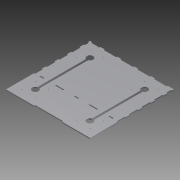
# Autodesk Inventor part: base top2
Saved by Autodesk Inventor 2011 (Build 150239000, 239)
## iProperties
Created: 2011-07-30
Part Number: base top2
Document SubType Name: Modeling
Designer: adowning
Density: 1 g/cm^3
Author: adowning
Autodesk Inventor part; units mm, degrees
(part 1 of 2)
ref_plane "YZ Plane" through (0, 0, 0) normal (1, 0, 0) x (0, 1, 0)
ref_plane "XZ Plane" through (0, 0, 0) normal (0, 1, 0) x (-1, 0, 0)
ref_plane "XY Plane" through (0, 0, 0) normal (0, 0, 1) x (1, 0, 0)
sketch "Sketch1" plane through (0, 0, 0) normal (0, 0, 1) x (1, 0, 0)
  point P0 (0, 0)
sketch "Sketch2" plane through (0, 0, 0) normal (0, 1, 0) x (-1, 0, 0)
  line L0 (74.6367, 49.7732) -> (-433.3633, 49.7732)
  line L1 (-433.3633, 49.7732) -> (-433.3633, -458.2268)
  line L2 (-433.3633, -458.2268) -> (74.6367, -458.2268)
  line L3 (74.6367, -458.2268) -> (74.6367, 49.7732)
  line L4 (74.6367, -458.2268) -> (-14.2633, -458.2268)
  line L5 (-14.2633, -382.0268) -> (-14.2633, -369.3268)
  line L6 (-14.2633, -369.3268) -> (-1.5633, -369.3268)
  line L7 (74.6367, -369.3268) -> (74.6367, -458.2268)
  line L8 (-433.3633, -458.2268) -> (-344.4633, -458.2268)
  line L9 (-344.4633, -382.0268) -> (-344.4633, -369.3268)
  line L10 (-344.4633, -369.3268) -> (-357.1633, -369.3268)
  line L11 (-433.3633, -369.3268) -> (-433.3633, -458.2268)
  line L12 (-433.3633, 49.7732) -> (-344.4633, 49.7732)
  line L13 (-344.4633, -26.4268) -> (-344.4633, -39.1268)
  line L14 (-344.4633, -39.1268) -> (-357.1633, -39.1268)
  line L15 (-433.3633, -39.1268) -> (-433.3633, 49.7732)
  line L16 (74.6367, 49.7732) -> (-14.2633, 49.7732)
  line L17 (-14.2633, -26.4268) -> (-14.2633, -39.1268)
  line L18 (-14.2633, -39.1268) -> (-1.5633, -39.1268)
  line L19 (74.6367, -39.1268) -> (74.6367, 49.7732)
  line L20 (74.6367, -458.2268) -> (26.0973, -458.2268)
  line L21 (26.0973, -411.6686) -> (26.0973, -409.6874)
  line L22 (26.0973, -409.6874) -> (28.0785, -409.6874)
  line L23 (74.6367, -409.6874) -> (74.6367, -458.2268)
  line L24 (-433.3633, 49.7732) -> (-384.8239, 49.7732)
  line L25 (-384.8239, 49.7732) -> (-384.8239, 5.3232)
  line L26 (-384.8239, 5.3232) -> (-433.3633, 5.3232)
  line L27 (-433.3633, 5.3232) -> (-433.3633, 49.7732)
  line L28 (74.6367, -458.2268) -> (-54.6239, -458.2268)
  line L29 (74.6367, -328.9662) -> (74.6367, -458.2268)
  line L30 (-433.3633, 49.7732) -> (-304.1027, 49.7732)
  line L31 (-433.3633, -79.4874) -> (-433.3633, 49.7732)
  line L32 (-433.3633, 49.7732) -> (-384.8239, 49.7732)
  line L33 (-384.8239, 1.2338) -> (-386.8051, 1.2338)
  line L34 (-433.3633, 1.2338) -> (-433.3633, 49.7732)
  circle A0 centre (26.0973, -409.6874) radius 1.9812
  circle A1 centre (-54.6239, -409.6874) radius 1.9812
  circle A2 centre (-54.6239, -328.9662) radius 1.9812
  circle A3 centre (26.0973, -328.9662) radius 1.9812
  circle A4 centre (-304.1027, -409.6874) radius 1.9812
  arc A5 (-386.8051, -409.6874) -> (-384.8239, -407.7062) centre (-384.8239, -409.6874) ccw
  circle A6 centre (-384.8239, -328.9662) radius 1.9812
  circle A7 centre (-304.1027, -328.9662) radius 1.9812
  circle A8 centre (-304.1027, -79.4874) radius 1.9812
  circle A9 centre (-384.8239, -79.4874) radius 1.9812
  circle A10 centre (-384.8239, 1.2338) radius 1.9812
  circle A11 centre (-304.1027, 1.2338) radius 1.9812
  circle A12 centre (26.0973, 1.2338) radius 1.9812
  circle A13 centre (26.0973, -79.4874) radius 1.9812
  circle A14 centre (-54.6239, -79.4874) radius 1.9812
  circle A15 centre (-54.6239, 1.2338) radius 1.9812
  circle A16 centre (-14.2633, -369.3268) radius 12.7
  circle A17 centre (-344.4633, -369.3268) radius 12.7
  circle A18 centre (-344.4633, -39.1268) radius 12.7
  circle A19 centre (-14.2633, -39.1268) radius 12.7
  line L35 (26.0973, -409.6874) -> (26.0973, -407.7062)
  line L36 (26.0973, -409.6874) -> (24.1161, -409.6874)
  line L37 (-54.6239, -328.9662) -> (-52.6427, -328.9662)
  line L38 (24.1161, -328.9662) -> (28.0785, -328.9662)
  line L39 (26.0973, -330.9474) -> (26.0973, -326.985)
  line L40 (-54.6239, -328.9662) -> (-54.6239, -326.985)
  line L41 (-54.6239, -411.6686) -> (-54.6239, -407.7062)
  line L42 (-54.6239, -330.9474) -> (-54.6239, -328.9662)
  line L43 (-54.6239, -328.9662) -> (-56.6051, -328.9662)
  line L44 (-52.6427, -409.6874) -> (-56.6051, -409.6874)
  line L45 (-302.1215, -409.6874) -> (-306.0839, -409.6874)
  line L46 (-382.8427, -409.6874) -> (-386.8051, -409.6874)
  line L47 (-384.8239, -407.7062) -> (-384.8239, -411.6686)
  line L48 (-302.1215, -328.9662) -> (-306.0839, -328.9662)
  line L49 (-382.8427, -328.9662) -> (-386.8051, -328.9662)
  line L50 (-384.8239, -326.985) -> (-384.8239, -330.9474)
  line L51 (-304.1027, -407.7062) -> (-304.1027, -411.6686)
  line L52 (-304.1027, -79.4874) -> (-304.1027, -81.4686)
  line L53 (-304.1027, -326.985) -> (-304.1027, -330.9474)
  line L54 (-384.8239, 1.2338) -> (-382.8427, 1.2338)
  line L55 (-384.8239, 1.2338) -> (-384.8239, -0.7474)
  line L56 (-384.8239, -77.5062) -> (-384.8239, -81.4686)
  line L57 (-304.1027, -79.4874) -> (-306.0839, -79.4874)
  line L58 (-382.8427, -79.4874) -> (-386.8051, -79.4874)
  line L59 (-384.8239, 49.7732) -> (-384.8239, 5.3232)
  line L60 (-384.8239, 3.215) -> (-384.8239, 1.2338)
  line L61 (-304.1027, 3.215) -> (-304.1027, -0.7474)
  line L62 (-304.1027, -77.5062) -> (-304.1027, -79.4874)
  line L63 (-306.0839, 1.2338) -> (-302.1215, 1.2338)
  line L64 (-304.1027, -79.4874) -> (-302.1215, -79.4874)
  line L65 (-56.6051, -79.4874) -> (-52.6427, -79.4874)
  line L66 (24.1161, -79.4874) -> (28.0785, -79.4874)
  line L67 (-54.6239, -81.4686) -> (-54.6239, -77.5062)
  line L68 (-54.6239, -0.7474) -> (-54.6239, 3.215)
  line L69 (-56.6051, 1.2338) -> (-52.6427, 1.2338)
  line L70 (24.1161, 1.2338) -> (28.0785, 1.2338)
  line L71 (26.0973, -81.4686) -> (26.0973, -77.5062)
  line L72 (26.0973, -0.7474) -> (26.0973, 3.215)
  point P0 (0, 0)
  dimension "d0" = 508
  dimension "d1" = 508
  dimension "d2" = 88.9
  dimension "d3" = 88.9
  dimension "d4" = 88.9
  dimension "d5" = 88.9
  dimension "d6" = 88.9
  dimension "d7" = 88.9
  dimension "d8" = 88.9
  dimension "d9" = 88.9
  dimension "d10" = 48.5394
  dimension "d11" = 48.5394
  dimension "d12" = 48.5394
  dimension "d13" = 129.2606
  dimension "d14" = 129.2606
  dimension "d15" = 129.2606
  dimension "d16" = 129.2606
  dimension "d17" = 48.5394
  dimension "d18" = 48.5394
  dimension "d19" = 3.9624
  dimension "d20" = 3.9624
  dimension "d21" = 3.9624
  dimension "d22" = 3.9624
  dimension "d23" = 3.9624
  dimension "d24" = 3.9624
  dimension "d25" = 3.9624
  dimension "d26" = 3.9624
  dimension "d27" = 3.9624
  dimension "d28" = 3.9624
  dimension "d29" = 3.9624
  dimension "d30" = 3.9624
  dimension "d31" = 3.9624
  dimension "d32" = 3.9624
  dimension "d33" = 3.9624
  dimension "d34" = 3.9624
  dimension "d35" = 25.4
  dimension "d36" = 25.4
  dimension "d37" = 25.4
  dimension "d38" = 25.4
  constraints: 146 end point, 72 point on circle, 53 perpendicular, 25 parallel, 24 midpoint, 20 centre point, 10 horizontal, 8 coincident
  measures "d0" distance of L2.end L1.end
  measures "d1" distance of L1.end L0.end
  measures "d2" distance of L5.end L7.start
  measures "d3" distance of L4.end L5.end
  measures "d4" distance of L11.start L9.end
  measures "d5" distance of L9.end L8.end
  measures "d6" distance of L13.end L15.start
  measures "d7" distance of L12.end L13.end
  measures "d8" distance of L19.start L17.end
  measures "d9" distance of L17.end L16.end
  measures "d10" distance of L21.end L23.start
  measures "d11" distance of L20.end L21.end
  measures "d12" distance of L25.end L26.end
  measures "d13" distance of L37.start L29.start
  measures "d14" distance of L28.end L37.start
  measures "d15" distance of L52.start L31.start
  measures "d16" distance of L30.end L52.start
  measures "d17" distance of L33.start L34.start
  measures "d18" distance of L32.end L33.start
  measures "d19" diameter of A0
  measures "d20" diameter of A1
  measures "d21" diameter of A2
  measures "d22" diameter of A3
  measures "d23" diameter of A4
  measures "d24" diameter of A5
  measures "d25" diameter of A6
  measures "d26" diameter of A7
  measures "d27" diameter of A8
  measures "d28" diameter of A9
  measures "d29" diameter of A10
  measures "d30" diameter of A11
  measures "d31" diameter of A12
  measures "d32" diameter of A13
  measures "d33" diameter of A14
  measures "d34" diameter of A15
  measures "d35" diameter of A16
  measures "d36" diameter of A17
  measures "d37" diameter of A18
  measures "d38" diameter of A19
extrude "Extrusion1" add sketch "Sketch2" along normal blind 12.7
sketch "Sketch3" plane through (0, 12.7, 0) normal (0, 1, 0) x (1, 0, 0)
  line L0 (-74.6367, -49.7732) -> (-74.6367, 458.2268) projected
  line L1 (433.3633, 458.2268) -> (433.3633, -49.7732) projected
  line L2 (-74.6367, 458.2268) -> (433.3633, 458.2268)
  line L3 (433.3633, 458.2268) -> (433.3633, 445.5268)
  line L4 (433.3633, 445.5268) -> (-74.6367, 445.5268)
  line L5 (-74.6367, 445.5268) -> (-74.6367, 458.2268)
  line L6 (433.3633, 445.5268) -> (-74.6367, 445.5268)
  line L7 (-74.6367, 445.5268) -> (-74.6367, 432.8268)
  line L8 (-74.6367, 432.8268) -> (433.3633, 432.8268)
  line L9 (433.3633, 432.8268) -> (433.3633, 445.5268)
  line L10 (433.3633, 432.8268) -> (407.9633, 432.8268)
  line L11 (407.9633, 432.8268) -> (407.9633, 445.5268)
  line L12 (407.9633, 445.5268) -> (433.3633, 445.5268)
  line L13 (433.3633, 445.5268) -> (433.3633, 432.8268)
  line L14 (407.9633, 432.8268) -> (369.8633, 432.8268)
  line L15 (369.8633, 432.8268) -> (369.8633, 445.5268)
  line L16 (369.8633, 445.5268) -> (407.9633, 445.5268)
  line L17 (407.9633, 445.5268) -> (407.9633, 432.8268)
  line L18 (369.8633, 432.8268) -> (344.4633, 432.8268)
  line L19 (344.4633, 432.8268) -> (344.4633, 445.5268)
  line L20 (344.4633, 445.5268) -> (369.8633, 445.5268)
  line L21 (369.8633, 445.5268) -> (369.8633, 432.8268)
  line L22 (344.4633, 432.8268) -> (306.3633, 432.8268)
  line L23 (306.3633, 432.8268) -> (306.3633, 445.5268)
  line L24 (306.3633, 445.5268) -> (344.4633, 445.5268)
  line L25 (344.4633, 445.5268) -> (344.4633, 432.8268)
  line L26 (306.3633, 432.8268) -> (280.9633, 432.8268)
  line L27 (280.9633, 432.8268) -> (280.9633, 445.5268)
  line L28 (280.9633, 445.5268) -> (306.3633, 445.5268)
  line L29 (306.3633, 445.5268) -> (306.3633, 432.8268)
  line L30 (280.9633, 445.5268) -> (242.8633, 445.5268)
  line L31 (242.8633, 445.5268) -> (242.8633, 432.8268)
  line L32 (242.8633, 432.8268) -> (280.9633, 432.8268)
  line L33 (280.9633, 432.8268) -> (280.9633, 445.5268)
  line L34 (242.8633, 432.8268) -> (217.4633, 432.8268)
  line L35 (217.4633, 432.8268) -> (217.4633, 445.5268)
  line L36 (217.4633, 445.5268) -> (242.8633, 445.5268)
  line L37 (242.8633, 445.5268) -> (242.8633, 432.8268)
  line L38 (217.4633, 445.5268) -> (179.3633, 445.5268)
  line L39 (179.3633, 445.5268) -> (179.3633, 432.8268)
  line L40 (179.3633, 432.8268) -> (217.4633, 432.8268)
  line L41 (217.4633, 432.8268) -> (217.4633, 445.5268)
  line L42 (179.3633, 432.8268) -> (153.9633, 432.8268)
  line L43 (153.9633, 432.8268) -> (153.9633, 445.5268)
  line L44 (153.9633, 445.5268) -> (179.3633, 445.5268)
  line L45 (179.3633, 445.5268) -> (179.3633, 432.8268)
  line L46 (153.9633, 432.8268) -> (115.8633, 432.8268)
  line L47 (115.8633, 432.8268) -> (115.8633, 445.5268)
  line L48 (115.8633, 445.5268) -> (153.9633, 445.5268)
  line L49 (153.9633, 445.5268) -> (153.9633, 432.8268)
  line L50 (115.8633, 432.8268) -> (90.4633, 432.8268)
  line L51 (90.4633, 432.8268) -> (90.4633, 445.5268)
  line L52 (90.4633, 445.5268) -> (115.8633, 445.5268)
  line L53 (115.8633, 445.5268) -> (115.8633, 432.8268)
  line L54 (90.4633, 432.8268) -> (52.3633, 432.8268)
  line L55 (52.3633, 432.8268) -> (52.3633, 445.5268)
  line L56 (52.3633, 445.5268) -> (90.4633, 445.5268)
  line L57 (90.4633, 445.5268) -> (90.4633, 432.8268)
  line L58 (52.3633, 432.8268) -> (26.9633, 432.8268)
  line L59 (26.9633, 432.8268) -> (26.9633, 445.5268)
  line L60 (26.9633, 445.5268) -> (52.3633, 445.5268)
  line L61 (52.3633, 445.5268) -> (52.3633, 432.8268)
  line L62 (26.9633, 432.8268) -> (-11.1367, 432.8268)
  line L63 (-11.1367, 432.8268) -> (-11.1367, 445.5268)
  line L64 (-11.1367, 445.5268) -> (26.9633, 445.5268)
  line L65 (26.9633, 445.5268) -> (26.9633, 432.8268)
  line L66 (-11.1367, 445.5268) -> (-36.5367, 445.5268)
  line L67 (-36.5367, 445.5268) -> (-36.5367, 432.8268)
  line L68 (-36.5367, 432.8268) -> (-11.1367, 432.8268)
  line L69 (-11.1367, 432.8268) -> (-11.1367, 445.5268)
  point P0 (0, 0)
  dimension "d41" = 12.7
  dimension "d42" = 12.7
  dimension "d43" = 25.4
  dimension "d44" = 38.1
  dimension "d45" = 25.4
  dimension "d46" = 38.1
  dimension "d47" = 25.4
  dimension "d48" = 38.1
  dimension "d49" = 25.4
  dimension "d50" = 38.1
  dimension "d51" = 25.4
  dimension "d52" = 38.1
  dimension "d53" = 25.4
  dimension "d54" = 38.1
  dimension "d55" = 25.4
  dimension "d56" = 38.1
  dimension "d57" = 25.4
  constraints: 134 end point, 33 parallel, 17 horizontal, 16 perpendicular, 4 point on line, 1 midpoint, 1 vertical, 15 other
  measures "d41" distance of L2.end L3.end
  measures "d42" distance of L7.end L7.start
  measures "d43" distance of L11.end L12.end
  measures "d44" distance of L15.end L16.end
  measures "d45" distance of L19.end L20.end
  measures "d46" distance of L23.end L24.end
  measures "d47" distance of L27.end L28.end
  measures "d48" distance of L32.end L31.end
  measures "d49" distance of L35.end L36.end
  measures "d50" distance of L40.end L39.end
  measures "d51" distance of L43.end L44.end
  measures "d52" distance of L47.end L48.end
  measures "d53" distance of L51.end L52.end
  measures "d54" distance of L55.end L56.end
  measures "d55" distance of L59.end L60.end
  measures "d56" distance of L63.end L64.end
  measures "d57" distance of L68.end L67.end
extrude "Extrusion2" cut sketch "Sketch3" against normal blind 25.4 contours L67 L4 L63 L8 | L59 L4 L55 L8 | L1 L8 L11 L4 | L51 L4 L47 L8 | L15 L8 L19 L4 | L43 L4 L39 L8 | L23 L8 L27 L4 | L35 L4 L31 L8
sketch "Sketch4" plane through (0, 12.7, 0) normal (0, 1, 0) x (1, 0, 0)
  line L0 (386.8051, 409.6874) -> (384.8239, 409.6874) projected
  line L1 (384.8239, 409.6874) -> (384.8239, 407.7062) projected
  arc A0 (386.8051, 409.6874) -> (384.8239, 407.7062) centre (384.8239, 409.6874) ccw projected
  circle A1 centre (384.8239, 409.6874) radius 1.9812
  point P0 (0, 0)
  constraints: 1 centre point, 1 coincident
extrude "Extrusion3" cut sketch "Sketch4" against normal blind 25.4 contours A1 L1 L0
sketch "Sketch5" plane through (0, 12.7, 0) normal (0, 1, 0) x (1, 0, 0)
  line L0 (433.3633, 432.8268) -> (407.9633, 432.8268) projected
  line L1 (407.9633, 432.8268) -> (407.9633, 445.5268) projected
  line L2 (407.9633, 445.5268) -> (433.3633, 445.5268) projected
  line L3 (433.3633, 432.8268) -> (433.3633, -49.7732) projected
  line L4 (433.3633, 445.5268) -> (433.3633, 432.8268)
  point P0 (0, 0)
  constraints: 2 end point, 1 collinear
extrude "Extrusion4" add sketch "Sketch5" against normal blind 12.7
sketch "Sketch6" plane through (0, 12.7, 0) normal (0, 1, 0) x (1, 0, 0)
  line L0 (217.4633, 445.5268) -> (242.8633, 445.5268) projected
  line L1 (242.8633, 445.5268) -> (242.8633, 432.8268) projected
  line L2 (242.8633, 432.8268) -> (217.4633, 432.8268) projected
  line L3 (217.4633, 432.8268) -> (217.4633, 445.5268) projected
  line L4 (-36.5367, 432.8268) -> (-36.5367, 445.5268) projected
  line L5 (-36.5367, 445.5268) -> (-11.1367, 445.5268) projected
  line L6 (-11.1367, 445.5268) -> (-11.1367, 432.8268) projected
  line L7 (-11.1367, 432.8268) -> (-36.5367, 432.8268) projected
  line L8 (115.8633, 445.5268) -> (115.8633, 432.8268) projected
  line L9 (115.8633, 432.8268) -> (90.4633, 432.8268) projected
  line L10 (90.4633, 432.8268) -> (90.4633, 445.5268) projected
  line L11 (90.4633, 445.5268) -> (115.8633, 445.5268) projected
  line L12 (52.3633, 445.5268) -> (52.3633, 432.8268) projected
  line L13 (52.3633, 432.8268) -> (26.9633, 432.8268) projected
  line L14 (26.9633, 432.8268) -> (26.9633, 445.5268) projected
  line L15 (26.9633, 445.5268) -> (52.3633, 445.5268) projected
  line L16 (179.3633, 445.5268) -> (179.3633, 432.8268) projected
  line L17 (179.3633, 432.8268) -> (153.9633, 432.8268) projected
  line L18 (153.9633, 432.8268) -> (153.9633, 445.5268) projected
  line L19 (153.9633, 445.5268) -> (179.3633, 445.5268) projected
  line L20 (306.3633, 432.8268) -> (280.9633, 432.8268) projected
  line L21 (280.9633, 432.8268) -> (280.9633, 445.5268) projected
  line L22 (280.9633, 445.5268) -> (306.3633, 445.5268) projected
  line L23 (306.3633, 445.5268) -> (306.3633, 432.8268) projected
  line L24 (369.8633, 445.5268) -> (369.8633, 432.8268) projected
  line L25 (369.8633, 432.8268) -> (344.4633, 432.8268) projected
  line L26 (344.4633, 432.8268) -> (344.4633, 445.5268) projected
  line L27 (344.4633, 445.5268) -> (369.8633, 445.5268) projected
  point P0 (0, 0)
extrude "Extrusion5" add sketch "Sketch6" against normal blind 12.7
sketch "Sketch7" plane through (0, 12.7, 0) normal (0, 1, 0) x (1, 0, 0)
  circle A0 centre (14.2633, 369.3268) radius 12.7 projected
  circle A1 centre (344.4633, 369.3268) radius 12.7 projected
  circle A2 centre (344.4633, 39.1268) radius 12.7 projected
  circle A3 centre (304.1027, 79.4874) radius 1.9812 projected
  circle A4 centre (-26.0973, 409.6874) radius 1.9812 projected
  circle A5 centre (54.6239, 79.4874) radius 1.9812 projected
  circle A6 centre (304.1027, 328.9662) radius 1.9812 projected
  circle A7 centre (304.1027, 409.6874) radius 1.9812 projected
  circle A8 centre (304.1027, -1.2338) radius 1.9812 projected
  circle A9 centre (384.8239, 79.4874) radius 1.9812 projected
  circle A10 centre (-26.0973, 79.4874) radius 1.9812 projected
  circle A11 centre (54.6239, -1.2338) radius 1.9812 projected
  circle A12 centre (-26.0973, 328.9662) radius 1.9812 projected
  line L0 (433.3633, 458.2268) -> (433.3633, -49.7732) projected
  line L1 (-74.6367, 458.2268) -> (433.3633, 458.2268) projected
  line L2 (-74.6367, -49.7732) -> (-74.6367, 458.2268) projected
  line L3 (433.3633, -49.7732) -> (-74.6367, -49.7732) projected
  circle A13 centre (54.6239, 409.6874) radius 1.9812 projected
  circle A14 centre (384.8239, 328.9662) radius 1.9812 projected
  circle A15 centre (384.8239, -1.2338) radius 1.9812 projected
  circle A16 centre (54.6239, 328.9662) radius 1.9812 projected
  circle A17 centre (-26.0973, -1.2338) radius 1.9812 projected
  circle A18 centre (384.8239, 409.6874) radius 1.9812 projected
  circle A19 centre (14.2633, 39.1268) radius 12.7 projected
  point P0 (0, 0)
extrude "Extrusion6" cut sketch "Sketch7" against normal blind 6.35
sketch "Sketch8" plane through (0, 6.35, 0) normal (0, 1, 0) x (1, 0, 0)
  line L0 (-74.6367, -49.7732) -> (-74.6367, 458.2268) projected
  line L1 (433.3633, -49.7732) -> (-74.6367, -49.7732) projected
  line L2 (433.3633, 458.2268) -> (433.3633, -49.7732) projected
  line L3 (-74.6367, -49.7732) -> (-74.6367, 204.2268)
  line L4 (-74.6367, 204.2268) -> (-74.6367, 270.2668)
  line L5 (-74.6367, 270.2668) -> (-74.6367, 138.1868)
  line L6 (-74.6367, -49.7732) -> (113.3233, -49.7732)
  line L7 (113.3233, -49.7732) -> (245.4033, -49.7732)
  line L8 (433.3633, -49.7732) -> (433.3633, 138.1868)
  line L9 (433.3633, 138.1868) -> (433.3633, 270.2668)
  line L10 (-74.6367, 138.1868) -> (-68.2867, 138.1868)
  line L11 (-68.2867, 138.1868) -> (-68.2867, 131.8368)
  line L12 (-68.2867, 131.8368) -> (-74.6367, 131.8368)
  line L13 (-74.6367, 131.8368) -> (-74.6367, 138.1868)
  line L14 (-74.6367, 270.2668) -> (-68.2867, 270.2668)
  line L15 (-68.2867, 270.2668) -> (-68.2867, 276.6168)
  line L16 (-68.2867, 276.6168) -> (-74.6367, 276.6168)
  line L17 (-74.6367, 276.6168) -> (-74.6367, 270.2668)
  line L18 (113.3233, -49.7732) -> (106.9733, -49.7732)
  line L19 (106.9733, -49.7732) -> (106.9733, -43.4232)
  line L20 (106.9733, -43.4232) -> (113.3233, -43.4232)
  line L21 (113.3233, -43.4232) -> (113.3233, -49.7732)
  line L22 (245.4033, -49.7732) -> (251.7533, -49.7732)
  line L23 (251.7533, -49.7732) -> (251.7533, -43.4232)
  line L24 (251.7533, -43.4232) -> (245.4033, -43.4232)
  line L25 (245.4033, -43.4232) -> (245.4033, -49.7732)
  line L26 (433.3633, 138.1868) -> (427.0133, 138.1868)
  line L27 (427.0133, 138.1868) -> (427.0133, 131.8368)
  line L28 (427.0133, 131.8368) -> (433.3633, 131.8368)
  line L29 (433.3633, 131.8368) -> (433.3633, 138.1868)
  line L30 (433.3633, 270.2668) -> (427.0133, 270.2668)
  line L31 (427.0133, 270.2668) -> (427.0133, 276.6168)
  line L32 (427.0133, 276.6168) -> (433.3633, 276.6168)
  line L33 (433.3633, 276.6168) -> (433.3633, 270.2668)
  point P0 (0, 0)
  dimension "d68" = 254
  dimension "d69" = 66.04
  dimension "d70" = 132.08
  dimension "d71" = 187.96
  dimension "d72" = 132.08
  dimension "d73" = 6.35
  dimension "d74" = 6.35
  dimension "d75" = 6.35
  dimension "d76" = 6.35
  dimension "d77" = 6.35
  dimension "d78" = 6.35
  dimension "d79" = 6.35
  dimension "d80" = 6.35
  dimension "d81" = 6.35
  dimension "d82" = 6.35
  dimension "d83" = 6.35
  dimension "d84" = 6.35
  constraints: 62 end point, 12 parallel, 6 horizontal, 6 perpendicular, 6 point on line, 1 midpoint
  measures "d68" distance of L0.start L3.end
  measures "d69" distance of L3.end L4.end
  measures "d70" distance of L4.end L5.end
  measures "d71" distance of L0.start L6.end
  measures "d72" distance of L6.end L7.end
  measures "d73" distance of L11.end L12.end
  measures "d74" distance of L10.end L11.end
  measures "d75" distance of L16.end L15.end
  measures "d76" distance of L15.end L14.end
  measures "d77" distance of L19.end L20.end
  measures "d78" distance of L18.end L19.end
  measures "d79" distance of L24.end L23.end
  measures "d80" distance of L23.end L22.end
  measures "d81" distance of L28.end L27.end
  measures "d82" distance of L27.end L26.end
  measures "d83" distance of L31.end L32.end
  measures "d84" distance of L30.end L31.end
extrude "Extrusion7" cut sketch "Sketch8" against normal blind 6.35
sketch "Sketch9" plane through (0, 6.35, 0) normal (0, 1, 0) x (1, 0, 0)
  line L0 (433.3633, 270.2668) -> (433.3633, 138.1868) projected
  line L1 (-74.6367, 138.1868) -> (-74.6367, 270.2668) projected
  line L2 (245.4033, -49.7732) -> (113.3233, -49.7732) projected
  line L3 (-74.6367, 138.1868) -> (-74.6367, 176.2868)
  line L4 (-74.6367, 270.2668) -> (-74.6367, 232.1668)
  line L5 (113.3233, -49.7732) -> (151.4233, -49.7732)
  line L6 (245.4033, -49.7732) -> (207.3033, -49.7732)
  line L7 (433.3633, 138.1868) -> (433.3633, 176.2868)
  line L8 (433.3633, 270.2668) -> (433.3633, 232.1668)
  line L9 (207.3033, -49.7732) -> (200.9533, -49.7732)
  line L10 (200.9533, -49.7732) -> (200.9533, -43.4232)
  line L11 (200.9533, -43.4232) -> (207.3033, -43.4232)
  line L12 (207.3033, -43.4232) -> (207.3033, -49.7732)
  line L13 (151.4233, -49.7732) -> (157.7733, -49.7732)
  line L14 (157.7733, -49.7732) -> (157.7733, -43.4232)
  line L15 (157.7733, -43.4232) -> (151.4233, -43.4232)
  line L16 (151.4233, -43.4232) -> (151.4233, -49.7732)
  line L17 (-74.6367, 176.2868) -> (-68.2867, 176.2868)
  line L18 (-68.2867, 176.2868) -> (-68.2867, 182.6368)
  line L19 (-68.2867, 182.6368) -> (-74.6367, 182.6368)
  line L20 (-74.6367, 182.6368) -> (-74.6367, 176.2868)
  line L21 (-74.6367, 232.1668) -> (-68.2867, 232.1668)
  line L22 (-68.2867, 232.1668) -> (-68.2867, 225.8168)
  line L23 (-68.2867, 225.8168) -> (-74.6367, 225.8168)
  line L24 (-74.6367, 225.8168) -> (-74.6367, 232.1668)
  line L25 (433.3633, 176.2868) -> (427.0133, 176.2868)
  line L26 (427.0133, 176.2868) -> (427.0133, 182.6368)
  line L27 (427.0133, 182.6368) -> (433.3633, 182.6368)
  line L28 (433.3633, 182.6368) -> (433.3633, 176.2868)
  line L29 (433.3633, 232.1668) -> (427.0133, 232.1668)
  line L30 (427.0133, 232.1668) -> (427.0133, 225.8168)
  line L31 (427.0133, 225.8168) -> (433.3633, 225.8168)
  line L32 (433.3633, 225.8168) -> (433.3633, 232.1668)
  point P0 (0, 0)
  dimension "d87" = 38.1
  dimension "d88" = 38.1
  dimension "d89" = 38.1
  dimension "d90" = 38.1
  dimension "d91" = 6.35
  dimension "d92" = 6.35
  dimension "d93" = 6.35
  dimension "d94" = 6.35
  dimension "d95" = 6.35
  dimension "d96" = 6.35
  dimension "d97" = 6.35
  dimension "d98" = 6.35
  dimension "d99" = 6.35
  dimension "d100" = 6.35
  dimension "d101" = 6.35
  constraints: 60 end point, 12 parallel, 6 horizontal, 6 perpendicular, 6 point on line
  measures "d87" distance of L1.start L3.end
  measures "d88" distance of L1.end L4.end
  measures "d89" distance of L2.end L5.end
  measures "d90" distance of L2.start L6.end
  measures "d91" distance of L10.end L11.end
  measures "d92" distance of L15.end L14.end
  measures "d93" distance of L14.end L13.end
  measures "d94" distance of L19.end L18.end
  measures "d95" distance of L18.end L17.end
  measures "d96" distance of L22.end L23.end
  measures "d97" distance of L21.end L22.end
  measures "d98" distance of L26.end L27.end
  measures "d99" distance of L25.end L26.end
  measures "d100" distance of L31.end L30.end
  measures "d101" distance of L30.end L29.end
extrude "Extrusion8" cut sketch "Sketch9" against normal blind 6.35
sketch "Sketch10" plane through (0, 6.35, 0) normal (0, 1, 0) x (1, 0, 0)
  line L0 (207.3033, -43.4232) -> (207.3033, -49.7732) projected
  line L1 (245.4033, -49.7732) -> (207.3033, -49.7732) projected
  line L2 (245.4033, -49.7732) -> (245.4033, -43.4232) projected
  line L3 (245.4033, -43.4232) -> (251.7533, -43.4232) projected
  line L4 (251.7533, -43.4232) -> (251.7533, -49.7732) projected
  line L5 (433.3633, -49.7732) -> (251.7533, -49.7732) projected
  line L6 (433.3633, 131.8368) -> (433.3633, -49.7732) projected
  line L7 (433.3633, 131.8368) -> (427.0133, 131.8368) projected
  line L8 (427.0133, 131.8368) -> (427.0133, 138.1868) projected
  line L9 (427.0133, 138.1868) -> (433.3633, 138.1868) projected
  line L10 (433.3633, 176.2868) -> (433.3633, 138.1868) projected
  line L11 (433.3633, 176.2868) -> (427.0133, 176.2868) projected
  line L12 (427.0133, 176.2868) -> (427.0133, 182.6368) projected
  line L13 (427.0133, 182.6368) -> (433.3633, 182.6368) projected
  line L14 (433.3633, 225.8168) -> (433.3633, 182.6368) projected
  line L15 (433.3633, 225.8168) -> (427.0133, 225.8168) projected
  line L16 (427.0133, 225.8168) -> (427.0133, 232.1668) projected
  line L17 (427.0133, 232.1668) -> (433.3633, 232.1668) projected
  line L18 (433.3633, 270.2668) -> (433.3633, 232.1668) projected
  line L19 (433.3633, 270.2668) -> (427.0133, 270.2668) projected
  line L20 (427.0133, 270.2668) -> (427.0133, 276.6168) projected
  line L21 (427.0133, 276.6168) -> (433.3633, 276.6168) projected
  line L22 (433.3633, 458.2268) -> (433.3633, 276.6168) projected
  line L23 (-74.6367, 458.2268) -> (433.3633, 458.2268) projected
  line L24 (-74.6367, 276.6168) -> (-74.6367, 458.2268) projected
  line L25 (-74.6367, 276.6168) -> (-68.2867, 276.6168) projected
  line L26 (-68.2867, 276.6168) -> (-68.2867, 270.2668) projected
  line L27 (-68.2867, 270.2668) -> (-74.6367, 270.2668) projected
  line L28 (-74.6367, 232.1668) -> (-74.6367, 270.2668) projected
  line L29 (-74.6367, 232.1668) -> (-68.2867, 232.1668) projected
  line L30 (-68.2867, 232.1668) -> (-68.2867, 225.8168) projected
  line L31 (-68.2867, 225.8168) -> (-74.6367, 225.8168) projected
  line L32 (-74.6367, 182.6368) -> (-74.6367, 225.8168) projected
  line L33 (-74.6367, 182.6368) -> (-68.2867, 182.6368) projected
  line L34 (-68.2867, 182.6368) -> (-68.2867, 176.2868) projected
  line L35 (-68.2867, 176.2868) -> (-74.6367, 176.2868) projected
  line L36 (-74.6367, 138.1868) -> (-74.6367, 176.2868) projected
  line L37 (-74.6367, 138.1868) -> (-68.2867, 138.1868) projected
  line L38 (-68.2867, 138.1868) -> (-68.2867, 131.8368) projected
  line L39 (-68.2867, 131.8368) -> (-74.6367, 131.8368) projected
  line L40 (-74.6367, -49.7732) -> (-74.6367, 131.8368) projected
  line L41 (106.9733, -49.7732) -> (-74.6367, -49.7732) projected
  line L42 (106.9733, -49.7732) -> (106.9733, -43.4232) projected
  line L43 (106.9733, -43.4232) -> (113.3233, -43.4232) projected
  line L44 (113.3233, -43.4232) -> (113.3233, -49.7732) projected
  line L45 (151.4233, -49.7732) -> (113.3233, -49.7732) projected
  line L46 (151.4233, -49.7732) -> (151.4233, -43.4232) projected
  line L47 (151.4233, -43.4232) -> (157.7733, -43.4232) projected
  line L48 (157.7733, -43.4232) -> (157.7733, -49.7732) projected
  line L49 (200.9533, -49.7732) -> (157.7733, -49.7732) projected
  line L50 (200.9533, -49.7732) -> (200.9533, -43.4232) projected
  line L51 (200.9533, -43.4232) -> (207.3033, -43.4232) projected
  line L52 (-68.2867, 138.1868) -> (-68.2867, 270.2668)
  line L53 (113.3233, -43.4232) -> (251.7533, -43.4232)
  line L54 (427.0133, 138.1868) -> (427.0133, 276.6168)
  point P0 (0, 0)
  constraints: 6 end point, 2 perpendicular, 1 parallel
extrude "Extrusion9" cut sketch "Sketch10" against normal blind 6.35 contours L53 L2 L1 L0 | L50 L49 L48 L53 | L46 L45 L44 L53 | L54 L11 L10 L9 | L54 L15 L14 L13 | L37 L36 L35 L52 | L54 L19 L18 L17 | L33 L32 L31 L52 | L29 L28 L27 L52
sketch "Sketch11" plane through (0, 6.35, 0) normal (0, 1, 0) x (1, 0, 0)
  line L0 (433.3633, 458.2268) -> (433.3633, 276.6168) projected
  line L1 (-74.6367, 458.2268) -> (433.3633, 458.2268) projected
  line L2 (-74.6367, 458.2268) -> (-49.2367, 458.2268)
  line L3 (-49.2367, 458.2268) -> (-23.8367, 458.2268)
  line L4 (-23.8367, 458.2268) -> (1.5633, 458.2268)
  line L5 (1.5633, 458.2268) -> (26.9633, 458.2268)
  line L6 (26.9633, 458.2268) -> (52.3633, 458.2268)
  line L7 (52.3633, 458.2268) -> (77.7633, 458.2268)
  line L8 (77.7633, 458.2268) -> (103.1633, 458.2268)
  line L9 (103.1633, 458.2268) -> (128.5633, 458.2268)
  line L10 (128.5633, 458.2268) -> (153.9633, 458.2268)
  line L11 (153.9633, 458.2268) -> (179.3633, 458.2268)
  line L12 (179.3633, 458.2268) -> (204.7633, 458.2268)
  line L13 (204.7633, 458.2268) -> (230.1633, 458.2268)
  line L14 (230.1633, 458.2268) -> (255.5633, 458.2268)
  line L15 (255.5633, 458.2268) -> (280.9633, 458.2268)
  line L16 (280.9633, 458.2268) -> (306.3633, 458.2268)
  line L17 (306.3633, 458.2268) -> (331.7633, 458.2268)
  line L18 (331.7633, 458.2268) -> (357.1633, 458.2268)
  line L19 (357.1633, 458.2268) -> (382.5633, 458.2268)
  line L20 (382.5633, 458.2268) -> (407.9633, 458.2268)
  line L21 (407.9633, 458.2268) -> (433.3633, 458.2268)
  line L22 (-49.2367, 458.2268) -> (-23.8367, 458.2268)
  line L23 (-23.8367, 458.2268) -> (-23.8367, 451.8768)
  line L24 (-23.8367, 451.8768) -> (-49.2367, 451.8768)
  line L25 (-49.2367, 451.8768) -> (-49.2367, 458.2268)
  line L26 (1.5633, 458.2268) -> (26.9633, 458.2268)
  line L27 (26.9633, 458.2268) -> (26.9633, 451.8768)
  line L28 (26.9633, 451.8768) -> (1.5633, 451.8768)
  line L29 (1.5633, 451.8768) -> (1.5633, 458.2268)
  line L30 (52.3633, 458.2268) -> (77.7633, 458.2268)
  line L31 (77.7633, 458.2268) -> (77.7633, 451.8768)
  line L32 (77.7633, 451.8768) -> (52.3633, 451.8768)
  line L33 (52.3633, 451.8768) -> (52.3633, 458.2268)
  line L34 (103.1633, 458.2268) -> (128.5633, 458.2268)
  line L35 (128.5633, 458.2268) -> (128.5633, 451.8768)
  line L36 (128.5633, 451.8768) -> (103.1633, 451.8768)
  line L37 (103.1633, 451.8768) -> (103.1633, 458.2268)
  line L38 (153.9633, 458.2268) -> (179.3633, 458.2268)
  line L39 (179.3633, 458.2268) -> (179.3633, 451.8768)
  line L40 (179.3633, 451.8768) -> (153.9633, 451.8768)
  line L41 (153.9633, 451.8768) -> (153.9633, 458.2268)
  line L42 (204.7633, 458.2268) -> (230.1633, 458.2268)
  line L43 (230.1633, 458.2268) -> (230.1633, 451.8768)
  line L44 (230.1633, 451.8768) -> (204.7633, 451.8768)
  line L45 (204.7633, 451.8768) -> (204.7633, 458.2268)
  line L46 (255.5633, 458.2268) -> (280.9633, 458.2268)
  line L47 (280.9633, 458.2268) -> (280.9633, 451.8768)
  line L48 (280.9633, 451.8768) -> (255.5633, 451.8768)
  line L49 (255.5633, 451.8768) -> (255.5633, 458.2268)
  line L50 (306.3633, 458.2268) -> (331.7633, 458.2268)
  line L51 (331.7633, 458.2268) -> (331.7633, 451.8768)
  line L52 (331.7633, 451.8768) -> (306.3633, 451.8768)
  line L53 (306.3633, 451.8768) -> (306.3633, 458.2268)
  line L54 (357.1633, 458.2268) -> (382.5633, 458.2268)
  line L55 (382.5633, 458.2268) -> (382.5633, 451.8768)
  line L56 (382.5633, 451.8768) -> (357.1633, 451.8768)
  line L57 (357.1633, 451.8768) -> (357.1633, 458.2268)
  line L58 (407.9633, 458.2268) -> (433.3633, 458.2268)
  line L59 (433.3633, 458.2268) -> (433.3633, 451.8768)
  line L60 (433.3633, 451.8768) -> (407.9633, 451.8768)
  line L61 (407.9633, 451.8768) -> (407.9633, 458.2268)
  point P0 (0, 0)
  dimension "d106" = 25.4
  dimension "d107" = 25.4
  dimension "d108" = 25.4
  dimension "d109" = 25.4
  dimension "d110" = 25.4
  dimension "d111" = 25.4
  dimension "d112" = 25.4
  dimension "d113" = 25.4
  dimension "d114" = 25.4
  dimension "d115" = 25.4
  dimension "d116" = 25.4
  dimension "d117" = 25.4
  dimension "d118" = 25.4
  dimension "d119" = 25.4
  dimension "d120" = 25.4
  dimension "d121" = 25.4
  dimension "d122" = 25.4
  dimension "d123" = 25.4
  dimension "d124" = 25.4
  dimension "d125" = 25.4
  dimension "d126" = 6.35
  constraints: 120 end point, 20 parallel, 11 horizontal, 10 perpendicular, 1 point on line, 20 other
  measures "d106" distance of L2.start L2.end
  measures "d107" distance of L2.end L3.end
  measures "d108" distance of L3.end L4.end
  measures "d109" distance of L4.end L5.end
  measures "d110" distance of L5.end L6.end
  measures "d111" distance of L6.end L7.end
  measures "d112" distance of L7.end L8.end
  measures "d113" distance of L8.end L9.end
  measures "d114" distance of L9.end L10.end
  measures "d115" distance of L10.end L11.end
  measures "d116" distance of L11.end L12.end
  measures "d117" distance of L12.end L13.end
  measures "d118" distance of L13.end L14.end
  measures "d119" distance of L14.end L15.end
  measures "d120" distance of L15.end L16.end
  measures "d121" distance of L16.end L17.end
  measures "d122" distance of L17.end L18.end
  measures "d123" distance of L18.end L19.end
  measures "d124" distance of L19.end L20.end
  measures "d125" distance of L20.end L0.start
  measures "d126" distance of L22.end L23.end
extrude "Extrusion10" cut sketch "Sketch11" against normal blind 25.4
sketch "Sketch12" plane through (0, 6.35, 0) normal (0, 1, 0) x (1, 0, 0)
  line L0 (-49.2367, 451.8768) -> (-49.2367, 458.2268) projected
  line L1 (-74.6367, 458.2268) -> (-49.2367, 458.2268) projected
  line L2 (-74.6367, 276.6168) -> (-74.6367, 458.2268) projected
  line L3 (357.1633, 451.8768) -> (357.1633, 458.2268) projected
  line L4 (331.7633, 458.2268) -> (357.1633, 458.2268) projected
  line L5 (331.7633, 458.2268) -> (331.7633, 451.8768) projected
  line L6 (255.5633, 451.8768) -> (255.5633, 458.2268) projected
  line L7 (230.1633, 458.2268) -> (255.5633, 458.2268) projected
  line L8 (230.1633, 458.2268) -> (230.1633, 451.8768) projected
  line L9 (153.9633, 451.8768) -> (153.9633, 458.2268) projected
  line L10 (128.5633, 458.2268) -> (153.9633, 458.2268) projected
  line L11 (128.5633, 458.2268) -> (128.5633, 451.8768) projected
  line L12 (52.3633, 451.8768) -> (52.3633, 458.2268) projected
  line L13 (26.9633, 458.2268) -> (52.3633, 458.2268) projected
  line L14 (26.9633, 458.2268) -> (26.9633, 451.8768) projected
  line L15 (-23.8367, 458.2268) -> (1.5633, 458.2268) projected
  line L16 (357.1633, 451.8768) -> (331.7633, 451.8768)
  line L17 (255.5633, 451.8768) -> (230.1633, 451.8768)
  line L18 (153.9633, 451.8768) -> (128.5633, 451.8768)
  line L19 (52.3633, 451.8768) -> (26.9633, 451.8768)
  line L20 (-49.2367, 451.8768) -> (-74.6367, 451.8768)
  point P0 (0, 0)
  constraints: 10 end point, 4 equal length, 1 perpendicular, 1 point on line
extrude "Extrusion11" cut sketch "Sketch12" against normal blind 25.4
sketch "Sketch13" plane through (0, 6.35, 0) normal (0, 1, 0) x (1, 0, 0)
  circle A0 centre (14.2633, 39.1268) radius 12.7 projected
  circle A1 centre (344.4633, 39.1268) radius 12.7 projected
  circle A2 centre (344.4633, 369.3268) radius 12.7 projected
  circle A3 centre (14.2633, 369.3268) radius 12.7 projected
  circle A4 centre (14.2633, 369.3268) radius 25.4
  circle A5 centre (344.4633, 369.3268) radius 25.4
  circle A6 centre (344.4633, 39.1268) radius 25.4
  circle A7 centre (14.2633, 39.1268) radius 25.4
  point P0 (0, 0)
  constraints: 4 centre point, 4 coincident
extrude "Extrusion12" cut sketch "Sketch13" against normal blind 25.4
sketch "Sketch14" plane through (0, 6.35, 0) normal (0, 1, 0) x (1, 0, 0)
  line L0 (-74.6367, 276.6168) -> (-74.6367, 451.8768) projected
  line L1 (-74.6367, 276.6168) -> (-68.2867, 276.6168) projected
  line L2 (-68.2867, 131.8368) -> (-74.6367, 131.8368) projected
  line L3 (-74.6367, -49.7732) -> (-74.6367, 131.8368) projected
  line L4 (106.9733, -49.7732) -> (-74.6367, -49.7732) projected
  line L5 (106.9733, -49.7732) -> (106.9733, -43.4232) projected
  line L6 (251.7533, -43.4232) -> (251.7533, -49.7732) projected
  line L7 (433.3633, -49.7732) -> (251.7533, -49.7732) projected
  line L8 (433.3633, 131.8368) -> (433.3633, -49.7732) projected
  line L9 (433.3633, 131.8368) -> (427.0133, 131.8368) projected
  line L10 (427.0133, 276.6168) -> (433.3633, 276.6168) projected
  line L11 (433.3633, 451.8768) -> (433.3633, 276.6168) projected
  line L12 (77.7633, 458.2268) -> (77.7633, 451.8768) projected
  line L13 (251.7533, -43.4232) -> (264.4533, -43.4232)
  line L14 (264.4533, -43.4232) -> (264.4533, -49.7732)
  line L15 (106.9733, -43.4232) -> (94.2733, -43.4232)
  line L16 (94.2733, -43.4232) -> (94.2733, -49.7732)
  line L17 (427.0133, 276.6168) -> (427.0133, 289.3168)
  line L18 (427.0133, 289.3168) -> (433.3633, 289.3168)
  line L19 (427.0133, 131.8368) -> (427.0133, 119.1368)
  line L20 (427.0133, 119.1368) -> (433.3633, 119.1368)
  line L21 (-68.2867, 276.6168) -> (-68.2867, 289.3168)
  line L22 (-74.6367, 289.3168) -> (-68.2867, 289.3168)
  line L23 (-68.2867, 131.8368) -> (-68.2867, 119.1368)
  line L24 (-68.2867, 119.1368) -> (-74.6367, 119.1368)
  point P0 (0, 0)
  dimension "d133" = 12.7
  dimension "d134" = 12.7
  dimension "d135" = 12.7
  dimension "d136" = 12.7
  constraints: 24 end point, 11 perpendicular, 6 point on line, 1 parallel
  measures "d133" distance of L6.start L13.end
  measures "d134" distance of L5.end L15.end
  measures "d135" distance of L10.start L17.end
  measures "d136" distance of L9.end L19.end
extrude "Extrusion13" cut sketch "Sketch14" against normal blind 25.4
sketch "Sketch15" plane through (0, 6.35, 0) normal (0, 1, 0) x (1, 0, 0)
  circle A0 centre (344.4633, 369.3268) radius 25.4 projected
  circle A1 centre (344.4633, 39.1268) radius 25.4 projected
  circle A2 centre (14.2633, 39.1268) radius 25.4 projected
  circle A3 centre (14.2633, 369.3268) radius 25.4 projected
  circle A4 centre (14.2633, 369.3268) radius 19.05
  circle A5 centre (344.4633, 369.3268) radius 19.05
  circle A6 centre (344.4633, 39.1268) radius 19.05
  circle A7 centre (14.2633, 39.1268) radius 19.05
  point P0 (0, 0)
  dimension "d139" = 38.1
  constraints: 4 centre point, 4 coincident
  measures "d139" diameter of A4
extrude "Extrusion14" add sketch "Sketch15" against normal blind 6.35
sketch "Sketch16" plane through (0, 6.35, 0) normal (0, 1, 0) x (1, 0, 0)
  circle A0 centre (14.2633, 369.3268) radius 19.05 projected
  circle A1 centre (344.4633, 369.3268) radius 19.05 projected
  line L0 (94.2733, -49.7732) -> (94.2733, -43.4232) projected
  line L1 (14.2633, 369.3268) -> (17.4383, 369.3268)
  line L2 (17.4383, 369.3268) -> (11.0883, 369.3268)
  line L3 (11.0883, 369.3268) -> (11.0883, 39.1268)
  line L4 (11.0883, 39.1268) -> (17.4383, 39.1268)
  line L5 (17.4383, 39.1268) -> (17.4383, 369.3268)
  line L6 (344.4633, 369.3268) -> (347.6383, 369.3268)
  line L7 (347.6383, 369.3268) -> (341.2883, 369.3268)
  line L8 (341.2883, 369.3268) -> (341.2883, 39.1268)
  line L9 (341.2883, 39.1268) -> (347.6383, 39.1268)
  line L10 (347.6383, 39.1268) -> (347.6383, 369.3268)
  point P0 (0, 0)
  dimension "d142" = 3.175
  dimension "d143" = 6.35
  dimension "d144" = 3.175
  dimension "d145" = 6.35
  constraints: 20 end point, 4 parallel, 4 perpendicular, 2 horizontal
  measures "d142" distance of L1.start L1.end
  measures "d143" distance of L4.end L3.end
  measures "d144" distance of L6.start L6.end
  measures "d145" distance of L9.end L8.end
extrude "Extrusion15" cut sketch "Sketch16" against normal blind 6.35 contours L3 L2 L1 L5 A0 | A0 L5 L4 L3 | A1 L10 L6 L7 L8 | L8 L7 L6 L10 A1 | A1 L10 L9 L8 picked at (12.1466, 363.0656)
fillet "Fillet1" radius 12.7 1 edges at (11.0883, 3.175, -350.5433)
fillet "Fillet2" radius 12.7 7 edges at (17.4383, 3.175, -350.5433) (341.2883, 3.175, -350.5433) (347.6383, 3.175, -350.5433) (341.2883, 3.175, -57.9104) (347.6383, 3.175, -57.9104) (11.0883, 3.175, -57.9104) (17.4383, 3.175, -57.9104)
sketch "Sketch17" plane through (0, 6.35, 0) normal (0, 1, 0) x (1, 0, 0)
  arc A0 (353.9883, 352.829) -> (334.9383, 352.829) centre (344.4633, 369.3268) ccw projected
  line L0 (94.2733, -49.7732) -> (94.2733, -43.4232) projected
  line L1 (344.4633, 369.3268) -> (350.8133, 369.3268)
  line L2 (350.8133, 369.3268) -> (338.1133, 369.3268)
  line L3 (338.1133, 369.3268) -> (338.1133, 39.1268)
  line L4 (338.1133, 39.1268) -> (350.8133, 39.1268)
  line L5 (350.8133, 39.1268) -> (350.8133, 369.3268)
  point P0 (0, 0)
  dimension "d150" = 6.35
  dimension "d151" = 12.7
  constraints: 10 end point, 2 parallel, 2 perpendicular, 1 horizontal
  measures "d150" distance of L1.start L1.end
  measures "d151" distance of L4.end L3.end
extrude "Extrusion16" cut sketch "Sketch17" against normal blind 25.4
sketch "Sketch18" plane through (0, 6.35, 0) normal (0, 1, 0) x (1, 0, 0)
  arc A0 (23.7883, 352.829) -> (4.7383, 352.829) centre (14.2633, 369.3268) ccw projected
  line L0 (17.4383, 341.8305) -> (17.4383, 66.6231) projected
  line L1 (14.2633, 369.3268) -> (20.6133, 369.3268)
  line L2 (20.6133, 369.3268) -> (7.9133, 369.3268)
  line L3 (7.9133, 369.3268) -> (7.9133, 39.1268)
  line L4 (7.9133, 39.1268) -> (20.6133, 39.1268)
  line L5 (20.6133, 39.1268) -> (20.6133, 369.3268)
  point P0 (0, 0)
  dimension "d154" = 6.35
  dimension "d155" = 12.7
  constraints: 10 end point, 2 parallel, 2 perpendicular, 1 horizontal
  measures "d154" distance of L1.start L1.end
  measures "d155" distance of L4.end L3.end
extrude "Extrusion17" cut sketch "Sketch18" against normal blind 25.4
sketch "Sketch19" plane through (0, 6.35, 0) normal (0, 1, 0) x (1, 0, 0)
  line L0 (427.0133, 289.3168) -> (433.3633, 289.3168)
  line L1 (433.3633, 289.3168) -> (433.3633, 125.4868)
  line L2 (433.3633, 125.4868) -> (427.0133, 125.4868)
  line L3 (427.0133, 125.4868) -> (427.0133, 289.3168)
  point P0 (0, 0)
  dimension "d158" = 163.83
  constraints: 8 end point, 2 parallel, 1 horizontal, 1 perpendicular
  measures "d158" distance of L0.end L1.end
extrude "Extrusion18" add sketch "Sketch19" against normal blind 6.35
sketch "Sketch20" plane through (0, 6.35, 0) normal (0, 1, 0) x (1, 0, 0)
  line L0 (433.3633, 451.8768) -> (433.3633, 125.4868) projected
  line L1 (433.3633, 451.8768) -> (427.0133, 451.8768)
  line L2 (427.0133, 451.8768) -> (427.0133, 420.1268)
  line L3 (427.0133, 420.1268) -> (433.3633, 420.1268)
  line L4 (433.3633, 420.1268) -> (433.3633, 451.8768)
  line L5 (427.0133, 420.1268) -> (433.3633, 420.1268)
  line L6 (433.3633, 420.1268) -> (433.3633, 394.7268)
  line L7 (433.3633, 394.7268) -> (427.0133, 394.7268)
  line L8 (427.0133, 394.7268) -> (427.0133, 420.1268)
  line L9 (427.0133, 394.7268) -> (433.3633, 394.7268)
  line L10 (433.3633, 394.7268) -> (433.3633, 343.9268)
  line L11 (433.3633, 343.9268) -> (427.0133, 343.9268)
  line L12 (427.0133, 343.9268) -> (427.0133, 394.7268)
  line L13 (427.0133, 343.9268) -> (433.3633, 343.9268)
  line L14 (433.3633, 343.9268) -> (433.3633, 318.5268)
  line L15 (433.3633, 318.5268) -> (427.0133, 318.5268)
  line L16 (427.0133, 318.5268) -> (427.0133, 343.9268)
  line L17 (427.0133, 318.5268) -> (433.3633, 318.5268)
  line L18 (433.3633, 318.5268) -> (433.3633, 267.7268)
  line L19 (433.3633, 267.7268) -> (427.0133, 267.7268)
  line L20 (427.0133, 267.7268) -> (427.0133, 318.5268)
  line L21 (427.0133, 267.7268) -> (433.3633, 267.7268)
  line L22 (433.3633, 267.7268) -> (433.3633, 242.3268)
  line L23 (433.3633, 242.3268) -> (427.0133, 242.3268)
  line L24 (427.0133, 242.3268) -> (427.0133, 267.7268)
  line L25 (427.0133, 242.3268) -> (433.3633, 242.3268)
  line L26 (433.3633, 242.3268) -> (433.3633, 191.5268)
  line L27 (433.3633, 191.5268) -> (427.0133, 191.5268)
  line L28 (427.0133, 191.5268) -> (427.0133, 242.3268)
  line L29 (427.0133, 191.5268) -> (433.3633, 191.5268)
  line L30 (433.3633, 191.5268) -> (433.3633, 166.1268)
  line L31 (433.3633, 166.1268) -> (427.0133, 166.1268)
  line L32 (427.0133, 166.1268) -> (427.0133, 191.5268)
  line L33 (427.0133, 166.1268) -> (433.3633, 166.1268)
  line L34 (433.3633, 166.1268) -> (433.3633, 125.4868)
  line L35 (433.3633, 125.4868) -> (427.0133, 125.4868)
  line L36 (427.0133, 125.4868) -> (427.0133, 166.1268)
  point P0 (0, 0)
  dimension "d161" = 31.75
  dimension "d162" = 25.4
  dimension "d163" = 50.8
  dimension "d164" = 25.4
  dimension "d165" = 50.8
  dimension "d166" = 25.4
  dimension "d167" = 50.8
  dimension "d168" = 25.4
  constraints: 72 end point, 18 parallel, 9 horizontal, 9 perpendicular, 8 other
  measures "d161" distance of L2.end L1.end
  measures "d162" distance of L5.end L6.end
  measures "d163" distance of L9.end L10.end
  measures "d164" distance of L13.end L14.end
  measures "d165" distance of L17.end L18.end
  measures "d166" distance of L21.end L22.end
  measures "d167" distance of L25.end L26.end
  measures "d168" distance of L29.end L30.end
extrude "Extrusion19" cut sketch "Sketch20" against normal blind 6.35 contours L0 L3 L2 L1 | L0 L11 L12 L7 | L0 L19 L20 L15 | L0 L27 L28 L23 | L0 L35 L36 L31
sketch "Sketch21" plane through (0, 6.35, 0) normal (0, 1, 0) x (1, 0, 0)
  line L0 (407.9633, 451.8768) -> (420.6633, 451.8768)
  line L1 (420.6633, 451.8768) -> (420.6633, 458.2268)
  line L2 (420.6633, 458.2268) -> (407.9633, 458.2268)
  line L3 (407.9633, 458.2268) -> (407.9633, 451.8768)
  line L4 (407.9633, 451.8768) -> (-74.6367, 451.8768)
  line L5 (-74.6367, 451.8768) -> (-74.6367, 458.2268)
  line L6 (-74.6367, 458.2268) -> (407.9633, 458.2268)
  line L7 (407.9633, 458.2268) -> (407.9633, 451.8768)
  line L8 (420.6633, 451.8768) -> (427.0133, 451.8768)
  line L9 (427.0133, 451.8768) -> (427.0133, 458.2268)
  line L10 (427.0133, 458.2268) -> (420.6633, 458.2268)
  line L11 (420.6633, 458.2268) -> (420.6633, 451.8768)
  point P0 (0, 0)
  dimension "d171" = 12.7
  constraints: 24 end point, 6 parallel, 3 horizontal, 3 perpendicular
  measures "d171" distance of L2.end L1.end
extrude "Extrusion20" add sketch "Sketch21" against normal blind 6.35
sketch "Sketch22" plane through (0, 6.35, 0) normal (0, 1, 0) x (1, 0, 0)
  line L0 (427.0133, 458.2268) -> (-74.6367, 458.2268) projected
  line L1 (427.0133, 458.2268) -> (420.6633, 458.2268)
  line L2 (420.6633, 458.2268) -> (420.6633, 451.8768)
  line L3 (420.6633, 451.8768) -> (427.0133, 451.8768)
  line L4 (427.0133, 451.8768) -> (427.0133, 458.2268)
  line L5 (420.6633, 451.8768) -> (395.2633, 451.8768)
  line L6 (395.2633, 451.8768) -> (395.2633, 458.2268)
  line L7 (395.2633, 458.2268) -> (420.6633, 458.2268)
  line L8 (420.6633, 458.2268) -> (420.6633, 451.8768)
  line L9 (395.2633, 451.8768) -> (319.0633, 451.8768)
  line L10 (319.0633, 451.8768) -> (319.0633, 458.2268)
  line L11 (319.0633, 458.2268) -> (395.2633, 458.2268)
  line L12 (395.2633, 458.2268) -> (395.2633, 451.8768)
  line L13 (319.0633, 451.8768) -> (293.6633, 451.8768)
  line L14 (293.6633, 451.8768) -> (293.6633, 458.2268)
  line L15 (293.6633, 458.2268) -> (319.0633, 458.2268)
  line L16 (319.0633, 458.2268) -> (319.0633, 451.8768)
  line L17 (293.6633, 451.8768) -> (217.4633, 451.8768)
  line L18 (217.4633, 451.8768) -> (217.4633, 458.2268)
  line L19 (217.4633, 458.2268) -> (293.6633, 458.2268)
  line L20 (293.6633, 458.2268) -> (293.6633, 451.8768)
  line L21 (217.4633, 451.8768) -> (192.0633, 451.8768)
  line L22 (192.0633, 451.8768) -> (192.0633, 458.2268)
  line L23 (192.0633, 458.2268) -> (217.4633, 458.2268)
  line L24 (217.4633, 458.2268) -> (217.4633, 451.8768)
  line L25 (192.0633, 451.8768) -> (115.8633, 451.8768)
  line L26 (115.8633, 451.8768) -> (115.8633, 458.2268)
  line L27 (115.8633, 458.2268) -> (192.0633, 458.2268)
  line L28 (192.0633, 458.2268) -> (192.0633, 451.8768)
  line L29 (115.8633, 451.8768) -> (90.4633, 451.8768)
  line L30 (90.4633, 451.8768) -> (90.4633, 458.2268)
  line L31 (90.4633, 458.2268) -> (115.8633, 458.2268)
  line L32 (115.8633, 458.2268) -> (115.8633, 451.8768)
  line L33 (90.4633, 451.8768) -> (14.2633, 451.8768)
  line L34 (14.2633, 451.8768) -> (14.2633, 458.2268)
  line L35 (14.2633, 458.2268) -> (90.4633, 458.2268)
  line L36 (90.4633, 458.2268) -> (90.4633, 451.8768)
  line L37 (14.2633, 451.8768) -> (-11.1367, 451.8768)
  line L38 (-11.1367, 451.8768) -> (-11.1367, 458.2268)
  line L39 (-11.1367, 458.2268) -> (14.2633, 458.2268)
  line L40 (14.2633, 458.2268) -> (14.2633, 451.8768)
  line L41 (-11.1367, 451.8768) -> (-74.6367, 451.8768)
  line L42 (-74.6367, 451.8768) -> (-74.6367, 458.2268)
  line L43 (-74.6367, 458.2268) -> (-11.1367, 458.2268)
  line L44 (-11.1367, 458.2268) -> (-11.1367, 451.8768)
  point P0 (0, 0)
  dimension "d174" = 6.35
  dimension "d175" = 6.35
  dimension "d176" = 25.4
  dimension "d177" = 76.2
  dimension "d178" = 25.4
  dimension "d179" = 76.2
  dimension "d180" = 25.4
  dimension "d181" = 76.2
  dimension "d182" = 25.4
  dimension "d183" = 76.2
  dimension "d184" = 25.4
  constraints: 88 end point, 22 parallel, 11 horizontal, 11 perpendicular, 10 other
  measures "d174" distance of L3.end L2.end
  measures "d175" distance of L2.end L1.end
  measures "d176" distance of L6.end L7.end
  measures "d177" distance of L10.end L11.end
  measures "d178" distance of L14.end L15.end
  measures "d179" distance of L18.end L19.end
  measures "d180" distance of L22.end L23.end
  measures "d181" distance of L26.end L27.end
  measures "d182" distance of L30.end L31.end
  measures "d183" distance of L34.end L35.end
  measures "d184" distance of L38.end L39.end
extrude "Extrusion21" cut sketch "Sketch22" against normal blind 6.35 contours L4 L3 L2 L0 | L6 L9 L10 L0 | L14 L17 L18 L0 | L22 L25 L26 L0 | L30 L33 L34 L0 | L38 L41 L42 L0